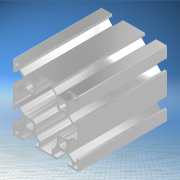
# Autodesk Inventor part: 60x60 aluminum
Saved by Autodesk Inventor 2020.2 (Build 242310000, 310)
## iProperties
Created: 2019-10-25
Part Number: 60x60 aluminum
Material: Aluminum 6061
Document SubType Name: Modeling
Designer: Sunoj
Density: 2.7 g/cm^3
Appearance: Aluminum - Flat
Mass: 1368.28 g
Surface Area: 5182.73 cm^2
Volume: 506.771 cm^3
Author: Sunoj
Autodesk Inventor part; units mm, degrees
ref_plane "YZ Plane" through (0, 0, 0) normal (1, 0, 0) x (0, 1, 0)
ref_plane "XZ Plane" through (0, 0, 0) normal (0, 1, 0) x (-1, 0, 0)
ref_plane "XY Plane" through (0, 0, 0) normal (0, 0, 1) x (1, 0, 0)
sketch "Sketch1" plane through (0, 0, 0) normal (0, 0, 1) x (1, 0, 0)
  line L0 (-15, -35.1) -> (-15, -44)
  line L1 (-15, -44) -> (-15, -35.1)
  line L2 (-14.9, -35) -> (-14.1, -35)
  line L3 (-14.9, -35) -> (-14.1, -35)
  arc A0 (-13, -34.85) -> (-13.1, -34.75) centre (-13.1, -34.85) ccw
  line L4 (-13.9, -34.75) -> (-13.1, -34.75)
  line L5 (-6, -34.75) -> (-6, -25.25)
  line L6 (-13, -21.75) -> (-9.5, -21.75)
  line L7 (-6, -25.25) -> (-9.5, -21.75)
  arc A1 (-13.1, -25.25) -> (-13, -25.15) centre (-13.1, -25.15) ccw
  line L8 (-13, -21.75) -> (-13, -25.15)
  line L9 (-13.1, -25.25) -> (-13.9, -25.25)
  arc A2 (-14, -25.15) -> (-13.9, -25.25) centre (-13.9, -25.15) ccw
  arc A3 (-14, -25.1) -> (-14.1, -25) centre (-14.1, -25.1) ccw
  arc A4 (-15, -24.9) -> (-14.9, -25) centre (-14.9, -24.9) ccw
  line L10 (-14.1, -25) -> (-14.9, -25)
  line L11 (-15, -24.9) -> (-15, -15)
  arc A5 (-15, -44) -> (-14, -45) centre (-14, -44) ccw
  arc A6 (-5.1, -45) -> (-5, -44.9) centre (-5.1, -44.9) ccw
  line L12 (-14, -45) -> (-5.1, -45)
  arc A7 (-4.9, -44) -> (-5, -44.1) centre (-4.9, -44.1) ccw
  line L13 (-5, -44.9) -> (-5, -44.1)
  arc A8 (-4.75, -43.1) -> (-4.75, -43.1) centre (-4.85, -43.1) ccw
  line L14 (-4.75, -43.9) -> (-4.75, -43.1)
  line L15 (-8.25, -43.1) -> (-4.75, -43.1)
  line L16 (-4.75, -43.1) -> (-8.25, -43.1)
  line L17 (8.25, -39.5) -> (4.75, -36)
  line L18 (4.85, -43) -> (8.25, -43)
  line L19 (8.25, -39.5) -> (8.25, -43)
  arc A9 (4.85, -43) -> (4.85, -43) centre (4.85, -43.1) ccw
  line L20 (4.85, -43) -> (4.85, -43.8)
  line L21 (4.85, -43) -> (4.85, -43.8)
  arc A10 (5.1, -44) -> (5, -43.9) centre (5, -44) ccw
  line L22 (4.95, -43.9) -> (5, -43.9)
  circle A11 centre (0, -30) radius 3.75
  circle A12 centre (0, -30) radius 3.75
  line L23 (-12.5503, -20.3) -> (-8.4723, -20.3)
  line L24 (-12.5503, -20.3) -> (-8.4723, -20.3)
  arc A13 (3.341, -24.4281) -> (5.5796, -26.6667) centre (15.0077, -15) ccw
  line L25 (9.7077, -38.48) -> (9.7077, -42.5)
  line L26 (9.7077, -38.48) -> (9.7077, -42.5)
  line L27 (15.0077, -15) -> (11.0077, -15)
  line L28 (15.0077, -15) -> (15.0077, -11)
  circle A14 centre (15.0077, -15) radius 4
  arc A15 (-15, -44) -> (-14, -45) centre (-14, -44) ccw
  arc A16 (-5.1, -45) -> (-5, -44.9) centre (-5.1, -44.9) ccw
  arc A17 (-4.85, -44) -> (-4.75, -43.9) centre (-4.85, -43.9) ccw
  line L29 (-4.75, -43.1) -> (-4.75, -43.9)
  arc A18 (-4.75, -43.1) -> (-4.75, -43.1) centre (-4.85, -43.1) ccw
  line L30 (-8.25, -43.1) -> (-8.25, -39.5)
  line L31 (-13, -38.25) -> (-9.5, -38.25)
  line L32 (-6, -34.75) -> (-6, -25.25)
  line L33 (-9.5, -21.75) -> (-13, -21.75)
  arc A19 (-13.1, -25.25) -> (-13, -25.15) centre (-13.1, -25.15) ccw
  line L34 (-13.9, -25.25) -> (-13.1, -25.25)
  arc A20 (-14, -25.15) -> (-13.9, -25.25) centre (-13.9, -25.15) ccw
  arc A21 (-14, -25.1) -> (-14.1, -25) centre (-14.1, -25.1) ccw
  arc A22 (-15, -24.9) -> (-14.9, -25) centre (-14.9, -24.9) ccw
  arc A23 (5.1, -44) -> (5, -43.9) centre (5, -44) ccw
  arc A24 (4.85, -43) -> (4.85, -43) centre (4.85, -43.1) ccw
  arc A25 (3.341, -24.4281) -> (5.5796, -26.6667) centre (15.0077, -15) ccw
  line L35 (4.75, -36) -> (8.25, -39.5)
  line L36 (4.85, -43) -> (8.25, -43)
  line L37 (-15, -24.9) -> (-15, -15)
  arc A26 (-8.4723, -20.3) -> (-5.2137, -23.5286) centre (0.0077, -15) ccw
  arc A27 (-8.4723, -20.3) -> (3.341, -24.4281) centre (0.0077, -15) ccw
  line L38 (5, -43.9) -> (4.95, -43.9)
  arc A28 (5.5796, -26.6667) -> (9.7077, -38.48) centre (15.0077, -30) ccw
  line L39 (-13.5, -40.7) -> (-13.5, -42.5)
  line L40 (-13.5, -42.5) -> (-13.5, -40.7)
  line L41 (-12.5, -39.7) -> (-10.7, -39.7)
  line L42 (-9.7, -40.7) -> (-9.7, -42.5)
  line L43 (-12.5, -43.5) -> (-10.7, -43.5)
  line L44 (-10.7, -43.5) -> (-12.5, -43.5)
  arc A29 (-9.7, -40.7) -> (-10.7, -39.7) centre (-10.7, -40.7) ccw
  arc A30 (-9.7, -40.7) -> (-10.7, -39.7) centre (-10.7, -40.7) ccw
  arc A31 (-12.5, -39.7) -> (-13.5, -40.7) centre (-12.5, -40.7) ccw
  arc A32 (-12.5, -39.7) -> (-13.5, -40.7) centre (-12.5, -40.7) ccw
  arc A33 (-13.5, -42.5) -> (-12.5, -43.5) centre (-12.5, -42.5) ccw
  arc A34 (-10.7, -43.5) -> (-9.7, -42.5) centre (-10.7, -42.5) ccw
  line L45 (-14, -25.1) -> (-14, -25.15)
  line L46 (-14, -25.1) -> (-14, -25.15)
  line L47 (15, -43.5) -> (10.7077, -43.5)
  arc A35 (9.7077, -42.5) -> (10.7077, -43.5) centre (10.7077, -42.5) ccw
  line L48 (5.1, -44) -> (5.1, -44.8)
  line L49 (5.1, -44) -> (5.1, -44.8)
  line L50 (5.1, -45) -> (15, -45)
  arc A36 (5.1, -44.8) -> (5.1, -45) centre (5.1, -44.9) ccw
  arc A37 (5.1, -44.8) -> (5.1, -45) centre (5.1, -44.9) ccw
  line L51 (-13.5, -15) -> (-13.5, -19.4166)
  arc A38 (-13.5, -19.4166) -> (-12.5503, -20.3) centre (-12.6143, -19.4166) ccw
  line L52 (-13.9, -34.75) -> (-13.9, -34.75)
  line L53 (-14, -34.85) -> (-14, -34.9)
  line L54 (-14.1, -35) -> (-14.1, -35)
  arc A39 (-13.9, -34.75) -> (-14, -34.85) centre (-13.9, -34.85) ccw
  arc A40 (-14.1, -35) -> (-14, -34.9) centre (-14.1, -34.9) ccw
  arc A41 (-14.9, -35) -> (-15, -35.1) centre (-14.9, -35.1) ccw
  line L55 (-13, -34.85) -> (-13, -38.25)
  line L56 (-9.5, -38.25) -> (-6, -34.75)
  line L57 (-8.25, -39.5) -> (-4.75, -36)
  line L58 (-4.75, -36) -> (4.75, -36)
  line L59 (-4.9, -44) -> (-4.85, -44)
  arc A42 (4.85, -43.8) -> (4.95, -43.9) centre (4.95, -43.8) ccw
  line L60 (42.5658, -20.3) -> (38.4877, -20.3)
  line L61 (42.5658, -20.3) -> (38.4877, -20.3)
  arc A43 (26.6744, -24.4281) -> (38.4877, -20.3) centre (30.0077, -15) ccw
  line L62 (43.0154, -21.75) -> (39.5154, -21.75)
  line L63 (39.5154, -21.75) -> (43.0154, -21.75)
  arc A44 (35.2291, -23.5286) -> (38.4877, -20.3) centre (30.0077, -15) ccw
  line L64 (36.0154, -25.25) -> (39.5154, -21.75)
  line L65 (43.0154, -21.75) -> (43.0154, -25.15)
  line L66 (45.0154, -24.9) -> (45.0154, -15)
  line L67 (45.0154, -24.9) -> (45.0154, -15)
  line L68 (44.9154, -35) -> (44.1154, -35)
  line L69 (44.9154, -35) -> (44.1154, -35)
  line L70 (45.0154, -35.1) -> (45.0154, -44)
  line L71 (45.0154, -44) -> (45.0154, -35.1)
  line L72 (43.9154, -34.75) -> (43.1154, -34.75)
  arc A45 (43.1154, -34.75) -> (43.0154, -34.85) centre (43.1154, -34.85) ccw
  arc A46 (43.5154, -40.7) -> (42.5154, -39.7) centre (42.5154, -40.7) ccw
  arc A47 (43.5154, -40.7) -> (42.5154, -39.7) centre (42.5154, -40.7) ccw
  line L73 (42.5154, -39.7) -> (40.7154, -39.7)
  line L74 (43.0154, -38.25) -> (39.5154, -38.25)
  arc A48 (40.7154, -39.7) -> (39.7154, -40.7) centre (40.7154, -40.7) ccw
  arc A49 (40.7154, -39.7) -> (39.7154, -40.7) centre (40.7154, -40.7) ccw
  arc A50 (34.7654, -43.9) -> (34.8654, -44) centre (34.8654, -43.9) ccw
  line L75 (34.7654, -43.9) -> (34.7654, -43.1)
  line L76 (34.7654, -43.1) -> (34.7654, -43.9)
  arc A51 (34.7654, -43.1) -> (34.7654, -43.1) centre (34.8654, -43.1) ccw
  arc A52 (34.7654, -43.1) -> (34.7654, -43.1) centre (34.8654, -43.1) ccw
  arc A53 (35.0154, -44.1) -> (34.9154, -44) centre (34.9154, -44.1) ccw
  line L77 (35.0154, -44.9) -> (35.0154, -44.1)
  arc A54 (35.0154, -44.9) -> (35.1154, -45) centre (35.1154, -44.9) ccw
  arc A55 (35.0154, -44.9) -> (35.1154, -45) centre (35.1154, -44.9) ccw
  line L78 (38.2654, -43.1) -> (34.7654, -43.1)
  line L79 (34.7654, -43.1) -> (38.2654, -43.1)
  line L80 (44.0154, -45) -> (35.1154, -45)
  line L81 (38.2654, -43.1) -> (38.2654, -39.5)
  arc A56 (39.7154, -42.5) -> (40.7154, -43.5) centre (40.7154, -42.5) ccw
  line L82 (39.7154, -40.7) -> (39.7154, -42.5)
  line L83 (42.5154, -43.5) -> (40.7154, -43.5)
  line L84 (40.7154, -43.5) -> (42.5154, -43.5)
  arc A57 (25.1654, -43) -> (25.1654, -43) centre (25.1654, -43.1) ccw
  line L85 (25.1654, -43) -> (25.1654, -43.8)
  line L86 (25.1654, -43) -> (25.1654, -43.8)
  line L87 (25.0654, -43.9) -> (25.0154, -43.9)
  line L88 (25.0154, -43.9) -> (25.0654, -43.9)
  line L89 (24.9154, -44) -> (24.9154, -44.8)
  arc A58 (25.1654, -43) -> (25.1654, -43) centre (25.1654, -43.1) ccw
  line L90 (24.9154, -44) -> (24.9154, -44.8)
  line L91 (21.7654, -39.5) -> (25.2654, -36)
  arc A59 (20.3077, -38.48) -> (24.4358, -26.6667) centre (15.0077, -30) ccw
  line L92 (25.2654, -36) -> (21.7654, -39.5)
  line L93 (25.1654, -43) -> (21.7654, -43)
  line L94 (21.7654, -39.5) -> (21.7654, -43)
  arc A60 (25.0154, -43.9) -> (24.9154, -44) centre (25.0154, -44) ccw
  arc A61 (25.0154, -43.9) -> (24.9154, -44) centre (25.0154, -44) ccw
  arc A62 (24.9154, -45) -> (24.9154, -44.8) centre (24.9154, -44.9) ccw
  arc A63 (24.9154, -45) -> (24.9154, -44.8) centre (24.9154, -44.9) ccw
  line L95 (25.1654, -43) -> (21.7654, -43)
  line L96 (24.9154, -45) -> (15.0154, -45)
  line L97 (15.0154, -43.5) -> (19.3077, -43.5)
  arc A64 (19.3077, -43.5) -> (20.3077, -42.5) centre (19.3077, -42.5) ccw
  line L98 (20.3077, -38.48) -> (20.3077, -42.5)
  line L99 (20.3077, -38.48) -> (20.3077, -42.5)
  arc A65 (43.0154, -25.15) -> (43.1154, -25.25) centre (43.1154, -25.15) ccw
  line L100 (43.1154, -25.25) -> (43.9154, -25.25)
  arc A66 (43.9154, -25.25) -> (44.0154, -25.15) centre (43.9154, -25.15) ccw
  arc A67 (44.1154, -25) -> (44.0154, -25.1) centre (44.1154, -25.1) ccw
  arc A68 (44.9154, -25) -> (45.0154, -24.9) centre (44.9154, -24.9) ccw
  line L101 (44.1154, -25) -> (44.9154, -25)
  arc A69 (44.9154, -25) -> (45.0154, -24.9) centre (44.9154, -24.9) ccw
  arc A70 (44.1154, -25) -> (44.0154, -25.1) centre (44.1154, -25.1) ccw
  line L102 (44.0154, -25.1) -> (44.0154, -25.15)
  line L103 (44.0154, -25.1) -> (44.0154, -25.15)
  arc A71 (43.9154, -25.25) -> (44.0154, -25.15) centre (43.9154, -25.15) ccw
  line L104 (43.9154, -25.25) -> (43.1154, -25.25)
  arc A72 (43.0154, -25.15) -> (43.1154, -25.25) centre (43.1154, -25.15) ccw
  arc A73 (24.4358, -26.6667) -> (26.6744, -24.4281) centre (15.0077, -15) ccw
  arc A74 (24.4358, -26.6667) -> (26.6744, -24.4281) centre (15.0077, -15) ccw
  line L105 (36.0154, -34.75) -> (36.0154, -25.25)
  line L106 (36.0154, -34.75) -> (36.0154, -25.25)
  circle A75 centre (30.0154, -30) radius 3.75
  circle A76 centre (30.0154, -30) radius 3.75
  arc A77 (44.0154, -45) -> (45.0154, -44) centre (44.0154, -44) ccw
  line L107 (43.5154, -40.7) -> (43.5154, -42.5)
  line L108 (43.5154, -42.5) -> (43.5154, -40.7)
  arc A78 (42.5154, -43.5) -> (43.5154, -42.5) centre (42.5154, -42.5) ccw
  arc A79 (44.0154, -45) -> (45.0154, -44) centre (44.0154, -44) ccw
  line L109 (43.5154, -15) -> (43.5154, -19.4166)
  arc A80 (42.5658, -20.3) -> (43.5154, -19.4166) centre (42.6297, -19.4166) ccw
  line L110 (43.9154, -34.75) -> (43.9154, -34.75)
  line L111 (44.0154, -34.85) -> (44.0154, -34.9)
  line L112 (44.1154, -35) -> (44.1154, -35)
  arc A81 (44.0154, -34.85) -> (43.9154, -34.75) centre (43.9154, -34.85) ccw
  arc A82 (44.0154, -34.9) -> (44.1154, -35) centre (44.1154, -34.9) ccw
  arc A83 (45.0154, -35.1) -> (44.9154, -35) centre (44.9154, -35.1) ccw
  line L113 (43.0154, -34.85) -> (43.0154, -38.25)
  line L114 (39.5154, -38.25) -> (36.0154, -34.75)
  line L115 (38.2654, -39.5) -> (34.7654, -36)
  line L116 (34.7654, -36) -> (25.2654, -36)
  line L117 (34.9154, -44) -> (34.8654, -44)
  arc A84 (25.0654, -43.9) -> (25.1654, -43.8) centre (25.0654, -43.8) ccw
  line L118 (15, -43.5) -> (15.0154, -43.5)
  line L119 (15, -45) -> (15.0154, -45)
  line L120 (42.5658, -9.7) -> (38.4877, -9.7)
  line L121 (42.5658, -9.7) -> (38.4877, -9.7)
  arc A85 (38.4877, -9.7) -> (26.6744, -5.5719) centre (30.0077, -15) ccw
  line L122 (43.0154, -8.25) -> (39.5154, -8.25)
  line L123 (39.5154, -8.25) -> (43.0154, -8.25)
  arc A86 (38.4877, -9.7) -> (35.2291, -6.4714) centre (30.0077, -15) ccw
  line L124 (36.0154, -4.75) -> (39.5154, -8.25)
  line L125 (43.0154, -8.25) -> (43.0154, -4.85)
  line L126 (45.0154, -5.1) -> (45.0154, -15)
  line L127 (45.0154, -5.1) -> (45.0154, -15)
  line L128 (44.9154, 5) -> (44.1154, 5)
  line L129 (44.9154, 5) -> (44.1154, 5)
  line L130 (45.0154, 5.1) -> (45.0154, 14)
  line L131 (45.0154, 14) -> (45.0154, 5.1)
  line L132 (43.9154, 4.75) -> (43.1154, 4.75)
  arc A87 (43.0154, 4.85) -> (43.1154, 4.75) centre (43.1154, 4.85) ccw
  arc A88 (42.5154, 9.7) -> (43.5154, 10.7) centre (42.5154, 10.7) ccw
  arc A89 (42.5154, 9.7) -> (43.5154, 10.7) centre (42.5154, 10.7) ccw
  line L133 (42.5154, 9.7) -> (40.7154, 9.7)
  line L134 (43.0154, 8.25) -> (39.5154, 8.25)
  arc A90 (39.7154, 10.7) -> (40.7154, 9.7) centre (40.7154, 10.7) ccw
  arc A91 (39.7154, 10.7) -> (40.7154, 9.7) centre (40.7154, 10.7) ccw
  arc A92 (34.8654, 14) -> (34.7654, 13.9) centre (34.8654, 13.9) ccw
  line L135 (34.7654, 13.9) -> (34.7654, 13.1)
  line L136 (34.7654, 13.1) -> (34.7654, 13.9)
  arc A93 (34.7654, 13.1) -> (34.7654, 13.1) centre (34.8654, 13.1) ccw
  arc A94 (34.7654, 13.1) -> (34.7654, 13.1) centre (34.8654, 13.1) ccw
  arc A95 (34.9154, 14) -> (35.0154, 14.1) centre (34.9154, 14.1) ccw
  line L137 (35.0154, 14.9) -> (35.0154, 14.1)
  arc A96 (35.1154, 15) -> (35.0154, 14.9) centre (35.1154, 14.9) ccw
  arc A97 (35.1154, 15) -> (35.0154, 14.9) centre (35.1154, 14.9) ccw
  line L138 (38.2654, 13.1) -> (34.7654, 13.1)
  line L139 (34.7654, 13.1) -> (38.2654, 13.1)
  line L140 (44.0154, 15) -> (35.1154, 15)
  line L141 (38.2654, 13.1) -> (38.2654, 9.5)
  arc A98 (40.7154, 13.5) -> (39.7154, 12.5) centre (40.7154, 12.5) ccw
  line L142 (39.7154, 10.7) -> (39.7154, 12.5)
  line L143 (42.5154, 13.5) -> (40.7154, 13.5)
  line L144 (40.7154, 13.5) -> (42.5154, 13.5)
  arc A99 (25.1654, 13) -> (25.1654, 13) centre (25.1654, 13.1) ccw
  line L145 (25.1654, 13) -> (25.1654, 13.8)
  line L146 (25.1654, 13) -> (25.1654, 13.8)
  line L147 (25.0654, 13.9) -> (25.0154, 13.9)
  line L148 (25.0154, 13.9) -> (25.0654, 13.9)
  line L149 (24.9154, 14) -> (24.9154, 14.8)
  arc A100 (25.1654, 13) -> (25.1654, 13) centre (25.1654, 13.1) ccw
  line L150 (24.9154, 14) -> (24.9154, 14.8)
  line L151 (21.7654, 9.5) -> (25.2654, 6)
  arc A101 (24.4358, -3.3333) -> (20.3077, 8.48) centre (15.0077, 0) ccw
  line L152 (25.2654, 6) -> (21.7654, 9.5)
  line L153 (25.1654, 13) -> (21.7654, 13)
  line L154 (21.7654, 9.5) -> (21.7654, 13)
  arc A102 (24.9154, 14) -> (25.0154, 13.9) centre (25.0154, 14) ccw
  arc A103 (24.9154, 14) -> (25.0154, 13.9) centre (25.0154, 14) ccw
  arc A104 (24.9154, 14.8) -> (24.9154, 15) centre (24.9154, 14.9) ccw
  arc A105 (24.9154, 14.8) -> (24.9154, 15) centre (24.9154, 14.9) ccw
  line L155 (25.1654, 13) -> (21.7654, 13)
  line L156 (24.9154, 15) -> (15.0154, 15)
  line L157 (15.0154, 13.5) -> (19.3077, 13.5)
  arc A106 (20.3077, 12.5) -> (19.3077, 13.5) centre (19.3077, 12.5) ccw
  line L158 (20.3077, 8.48) -> (20.3077, 12.5)
  line L159 (20.3077, 8.48) -> (20.3077, 12.5)
  arc A107 (43.1154, -4.75) -> (43.0154, -4.85) centre (43.1154, -4.85) ccw
  line L160 (43.1154, -4.75) -> (43.9154, -4.75)
  arc A108 (44.0154, -4.85) -> (43.9154, -4.75) centre (43.9154, -4.85) ccw
  arc A109 (44.0154, -4.9) -> (44.1154, -5) centre (44.1154, -4.9) ccw
  arc A110 (45.0154, -5.1) -> (44.9154, -5) centre (44.9154, -5.1) ccw
  line L161 (44.1154, -5) -> (44.9154, -5)
  arc A111 (45.0154, -5.1) -> (44.9154, -5) centre (44.9154, -5.1) ccw
  arc A112 (44.0154, -4.9) -> (44.1154, -5) centre (44.1154, -4.9) ccw
  line L162 (44.0154, -4.9) -> (44.0154, -4.85)
  line L163 (44.0154, -4.9) -> (44.0154, -4.85)
  arc A113 (44.0154, -4.85) -> (43.9154, -4.75) centre (43.9154, -4.85) ccw
  line L164 (43.9154, -4.75) -> (43.1154, -4.75)
  arc A114 (43.1154, -4.75) -> (43.0154, -4.85) centre (43.1154, -4.85) ccw
  arc A115 (26.6744, -5.5719) -> (24.4358, -3.3333) centre (15.0077, -15) ccw
  arc A116 (26.6744, -5.5719) -> (24.4358, -3.3333) centre (15.0077, -15) ccw
  line L165 (36.0154, 4.75) -> (36.0154, -4.75)
  line L166 (36.0154, 4.75) -> (36.0154, -4.75)
  circle A117 centre (30.0154, 0) radius 3.75
  circle A118 centre (30.0154, 0) radius 3.75
  arc A119 (45.0154, 14) -> (44.0154, 15) centre (44.0154, 14) ccw
  line L167 (43.5154, 10.7) -> (43.5154, 12.5)
  line L168 (43.5154, 12.5) -> (43.5154, 10.7)
  arc A120 (43.5154, 12.5) -> (42.5154, 13.5) centre (42.5154, 12.5) ccw
  arc A121 (45.0154, 14) -> (44.0154, 15) centre (44.0154, 14) ccw
  line L169 (43.5154, -15) -> (43.5154, -10.5834)
  arc A122 (43.5154, -10.5834) -> (42.5658, -9.7) centre (42.6297, -10.5834) ccw
  line L170 (43.9154, 4.75) -> (43.9154, 4.75)
  line L171 (44.0154, 4.85) -> (44.0154, 4.9)
  line L172 (44.1154, 5) -> (44.1154, 5)
  arc A123 (43.9154, 4.75) -> (44.0154, 4.85) centre (43.9154, 4.85) ccw
  arc A124 (44.1154, 5) -> (44.0154, 4.9) centre (44.1154, 4.9) ccw
  arc A125 (44.9154, 5) -> (45.0154, 5.1) centre (44.9154, 5.1) ccw
  line L173 (43.0154, 4.85) -> (43.0154, 8.25)
  line L174 (39.5154, 8.25) -> (36.0154, 4.75)
  line L175 (38.2654, 9.5) -> (34.7654, 6)
  line L176 (34.7654, 6) -> (25.2654, 6)
  line L177 (34.9154, 14) -> (34.8654, 14)
  arc A126 (25.1654, 13.8) -> (25.0654, 13.9) centre (25.0654, 13.8) ccw
  line L178 (-13.9, -4.75) -> (-13.1, -4.75)
  arc A127 (-13.9, -4.75) -> (-14, -4.85) centre (-13.9, -4.85) ccw
  line L179 (-14, -4.9) -> (-14, -4.85)
  line L180 (-14, -4.9) -> (-14, -4.85)
  arc A128 (-13, -4.85) -> (-13.1, -4.75) centre (-13.1, -4.85) ccw
  line L181 (-13, -8.25) -> (-13, -4.85)
  line L182 (-13, -8.25) -> (-9.5, -8.25)
  line L183 (-9.5, -8.25) -> (-13, -8.25)
  line L184 (-6, -4.75) -> (-9.5, -8.25)
  arc A129 (-5.2137, -6.4714) -> (-8.4723, -9.7) centre (0.0077, -15) ccw
  line L185 (-12.5503, -9.7) -> (-8.4723, -9.7)
  line L186 (-12.5503, -9.7) -> (-8.4723, -9.7)
  arc A130 (-12.5503, -9.7) -> (-13.5, -10.5834) centre (-12.6143, -10.5834) ccw
  line L187 (-15, -5.1) -> (-15, -15)
  line L188 (-15, -5.1) -> (-15, -15)
  line L189 (-13.5, -15) -> (-13.5, -10.5834)
  line L190 (-13.9, 4.75) -> (-13.9, 4.75)
  arc A131 (-14, 4.85) -> (-13.9, 4.75) centre (-13.9, 4.85) ccw
  line L191 (-13, 8.25) -> (-9.5, 8.25)
  line L192 (-12.5, 9.7) -> (-10.7, 9.7)
  line L193 (-13.5, 12.5) -> (-13.5, 10.7)
  line L194 (-13.5, 10.7) -> (-13.5, 12.5)
  line L195 (-15, 5.1) -> (-15, 14)
  line L196 (-15, 14) -> (-15, 5.1)
  arc A132 (-13.5, 10.7) -> (-12.5, 9.7) centre (-12.5, 10.7) ccw
  arc A133 (-13.5, 10.7) -> (-12.5, 9.7) centre (-12.5, 10.7) ccw
  line L197 (-14.9, 5) -> (-14.1, 5)
  line L198 (-14.9, 5) -> (-14.1, 5)
  line L199 (-13, 4.85) -> (-13, 8.25)
  line L200 (-9.5, 8.25) -> (-6, 4.75)
  line L201 (-8.25, 9.5) -> (-4.75, 6)
  arc A134 (-10.7, 9.7) -> (-9.7, 10.7) centre (-10.7, 10.7) ccw
  arc A135 (-10.7, 9.7) -> (-9.7, 10.7) centre (-10.7, 10.7) ccw
  line L202 (-9.7, 10.7) -> (-9.7, 12.5)
  line L203 (-8.25, 13.1) -> (-8.25, 9.5)
  line L204 (-8.25, 13.1) -> (-4.75, 13.1)
  line L205 (-4.75, 13.1) -> (-8.25, 13.1)
  line L206 (-4.9, 14) -> (-4.85, 14)
  arc A136 (-5, 14.1) -> (-4.9, 14) centre (-4.9, 14.1) ccw
  line L207 (-5, 14.9) -> (-5, 14.1)
  arc A137 (-5, 14.9) -> (-5.1, 15) centre (-5.1, 14.9) ccw
  arc A138 (-5, 14.9) -> (-5.1, 15) centre (-5.1, 14.9) ccw
  line L208 (-14.1, 5) -> (-14.1, 5)
  arc A139 (-15, 5.1) -> (-14.9, 5) centre (-14.9, 5.1) ccw
  arc A140 (-14, 4.9) -> (-14.1, 5) centre (-14.1, 4.9) ccw
  line L209 (9.7077, 8.48) -> (9.7077, 12.5)
  line L210 (9.7077, 8.48) -> (9.7077, 12.5)
  line L211 (8.25, 9.5) -> (8.25, 13)
  line L212 (4.85, 13) -> (8.25, 13)
  line L213 (4.85, 13) -> (8.25, 13)
  line L214 (5.1, 14) -> (5.1, 14.8)
  line L215 (5.1, 14) -> (5.1, 14.8)
  arc A141 (5.1, 15) -> (5.1, 14.8) centre (5.1, 14.9) ccw
  arc A142 (5.1, 15) -> (5.1, 14.8) centre (5.1, 14.9) ccw
  line L216 (4.95, 13.9) -> (5, 13.9)
  line L217 (5, 13.9) -> (4.95, 13.9)
  line L218 (5.1, 15) -> (15, 15)
  arc A143 (10.7077, 13.5) -> (9.7077, 12.5) centre (10.7077, 12.5) ccw
  line L219 (15, 13.5) -> (10.7077, 13.5)
  arc A144 (3.341, -5.5719) -> (-8.4723, -9.7) centre (0.0077, -15) ccw
  circle A145 centre (0, 0) radius 3.75
  circle A146 centre (0, 0) radius 3.75
  arc A147 (5.5796, -3.3333) -> (3.341, -5.5719) centre (15.0077, -15) ccw
  line L220 (8.25, 9.5) -> (4.75, 6)
  line L221 (4.75, 6) -> (8.25, 9.5)
  arc A148 (9.7077, 8.48) -> (5.5796, -3.3333) centre (15.0077, 0) ccw
  line L222 (-12.5, 13.5) -> (-10.7, 13.5)
  line L223 (-10.7, 13.5) -> (-12.5, 13.5)
  arc A149 (-9.7, 12.5) -> (-10.7, 13.5) centre (-10.7, 12.5) ccw
  arc A150 (-12.5, 13.5) -> (-13.5, 12.5) centre (-12.5, 12.5) ccw
  arc A151 (-14, 15) -> (-15, 14) centre (-14, 14) ccw
  arc A152 (-14, 15) -> (-15, 14) centre (-14, 14) ccw
  line L224 (-14, 15) -> (-5.1, 15)
  arc A153 (-4.75, 13.1) -> (-4.75, 13.1) centre (-4.85, 13.1) ccw
  arc A154 (-4.75, 13.1) -> (-4.75, 13.1) centre (-4.85, 13.1) ccw
  line L225 (-4.75, 13.9) -> (-4.75, 13.1)
  line L226 (-4.75, 13.1) -> (-4.75, 13.9)
  arc A155 (-4.75, 13.9) -> (-4.85, 14) centre (-4.85, 13.9) ccw
  arc A156 (4.85, 13) -> (4.85, 13) centre (4.85, 13.1) ccw
  line L227 (4.85, 13) -> (4.85, 13.8)
  line L228 (4.85, 13) -> (4.85, 13.8)
  arc A157 (4.85, 13) -> (4.85, 13) centre (4.85, 13.1) ccw
  arc A158 (5, 13.9) -> (5.1, 14) centre (5, 14) ccw
  arc A159 (4.95, 13.9) -> (4.85, 13.8) centre (4.95, 13.8) ccw
  line L229 (-4.75, 6) -> (4.75, 6)
  arc A160 (5, 13.9) -> (5.1, 14) centre (5, 14) ccw
  arc A161 (-13, -4.85) -> (-13.1, -4.75) centre (-13.1, -4.85) ccw
  line L230 (-13.1, -4.75) -> (-13.9, -4.75)
  arc A162 (-13.9, -4.75) -> (-14, -4.85) centre (-13.9, -4.85) ccw
  line L231 (-13.9, 4.75) -> (-13.1, 4.75)
  arc A163 (-13.1, 4.75) -> (-13, 4.85) centre (-13.1, 4.85) ccw
  line L232 (-6, 4.75) -> (-6, -4.75)
  line L233 (-6, 4.75) -> (-6, -4.75)
  arc A164 (-14.1, -5) -> (-14, -4.9) centre (-14.1, -4.9) ccw
  arc A165 (-14.9, -5) -> (-15, -5.1) centre (-14.9, -5.1) ccw
  line L234 (-14, 4.85) -> (-14, 4.9)
  arc A166 (5.5796, -3.3333) -> (3.341, -5.5719) centre (15.0077, -15) ccw
  arc A167 (-14.1, -5) -> (-14, -4.9) centre (-14.1, -4.9) ccw
  line L235 (-14.1, -5) -> (-14.9, -5)
  arc A168 (-14.9, -5) -> (-15, -5.1) centre (-14.9, -5.1) ccw
  line L236 (15.0154, 13.5) -> (15, 13.5)
  line L237 (15.0154, 15) -> (15, 15)
  point P0 (0, 0)
  point P1 (15, -30)
  point P2 (15, -30)
  point P3 (-14, -34.75)
  point P4 (15.0154, -30)
  point P5 (15.0154, -30)
  point P6 (44.0154, -34.75)
  point P7 (15.0154, 0)
  point P8 (15.0154, 0)
  point P9 (44.0154, 4.75)
  point P10 (-14, 4.75)
  point P11 (15, 0)
  point P12 (15, 0)
  point P13 (-5.2137, -6.4714)
  point P14 (5.5796, -3.3333)
  point P15 (24.4358, -26.6667)
  dimension "d0" = 9.9
  dimension "d1" = 4
  dimension "d2" = 4
  dimension "d3" = 0.1
  dimension "d4" = 0.1
  dimension "d5" = 9.9
  dimension "d6" = 0.1
  dimension "d7" = 0.1
  constraints: 476 end point, 324 point on circle, 168 centre point, 113 symmetric about line, 58 tangent, 16 point on line, 14 equal length, 12 equal radius, 12 vertical, 11 coincident, 11 horizontal, 11 perpendicular, 1 vertical alignment, 44 other
  measures "d0" distance of L11.start L11.end
  measures "d1" distance of L27.start L27.end
  measures "d2" distance of L27.start L28.end
  measures "d3" distance of L4.start point (-14, -34.75)
  measures "d4" radius of A39
  measures "d5" distance of L126.start L126.end
  measures "d6" distance of L132.start point (44.015, 4.75)
  measures "d7" radius of A123
extrude "Extrusion1" add sketch "Sketch1" along normal blind 80 contours A41 L2 A40 L53 A39 L4 A0 L55 L31 L56 L5 L7 L6 L8 A1 L9 A2 L45 A3 L10 A4 L11 L187 A165 L235 A164 L179 A127 L178 A128 L181 L182 L184 L232 L200 L191 L199 A163 L231 A131 L234 A140 L197 A139 L195 A151 L224 A137 L207 A136 L206 A155 L225 A153 L204 L203 L201 L229 L220 L211 L212 A156 L227 A159 L216 A158 L214 A141 L218 L237 L156 A104 L149 A102 L147 A126 L145 A99 L153 L154 L151 L176 L175 L141 L138 A93 L135 A92 L177 A95 L137 A96 L140 A119 L130 A125 L128 A124 L171 A123 L132 A87 L173 L134 L174 L165 L124 L122 L125 A107 L160 A108 L162 A109 L161 A110 L126 L66 A68 L101 A67 L102 A66 L100 A65 L65 L62 L64 L105 L114 L74 L113 A45 L72 A81 L111 A82 L68 A83 L70 A77 L80 A54 L77 A53 L117 A50 L75 A51 L78 L81 L115 L116 L91 L94 L93 A57 L85 A84 L87 A60 L89 A62 L96 L119 L50 A36 L48 A10 L22 A42 L20 A9 L18 L19 L17 L58 L57 L30 L15 A8 L14 A17 L59 A7 L13 A6 L12 A5 L0 | A8 L15 | A9 L20 | A57 L85 | A51 L78 | L204 A153 | L227 A156 | L145 A99 | L138 A93 picked at (-4.88, -43.1145) picked at (4.8863, -43.1261) picked at (25.1509, -43.07) picked at (34.8354, -43.1145) picked at (-4.8426, 13.1325) picked at (4.9044, 13.0775) picked at (25.1509, 13.07) picked at (34.8954, 13.1145)
body "Solid1"
